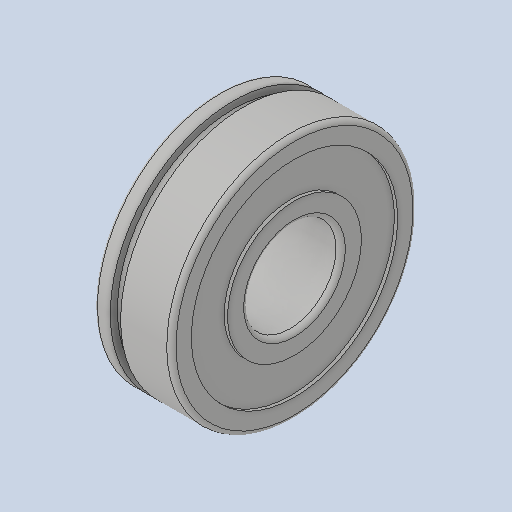
# Autodesk Inventor part: bearingB6201ZZNR
Saved by Autodesk Inventor 2025.2 (Build 292293000, 293)
## iProperties
Category: PARTsolutions
Company: MISUMI
Created: 2023-12-27
Part Number: bearingB6201ZZNR
Material: Generic
Catalog Web Link: www.cadenas.de
Description: bearing_b-Deep Groove Ball Bearings - Shield_b
Vendor: MISUMI
Document SubType Name: Modeling
Designer: psAdmin
Manufacturer: MISUMI
Mass: 6.48991 g
Surface Area: 29.9514 cm^2
Volume: 6.48991 cm^3
Density: 1 g/cm^3
Appearance: PSOLRGB-175-175-175
PSOL_IDENT_0: {$CADENAS_DATA/23d-libs/misumi/metric/12_bearing_holders/b6700zz.prj},175 {VTYP=3D},{NB=bearingB6201
PSOL_IDENT_1: ZZNR},{LINA=B6201ZZNR},{NN=bearing_b},{DATE=06.04.2023 02:22:35},{GEOMDATE=28.11.2013 13:02:00},{VER
PSOL_IDENT_2: SION=},{LINEID=100},{WBVAR=TS,TYS},{WBNUMERIC=}  {NB=bearingB6201ZZNR},{LINA=B6201ZZNR},{KT=DUMMY},{
PSOL_IDENT_3: PN=B6201ZZNR},{TS=},{TS1= '', 'Steel', 'S', 'Stainless Steel'},{TYS=NR},{TYS1=  '','w/o Retaining Ri
PSOL_IDENT_4: ng','NR','With Retaining Ring'},{MAT=52100 Bearing Steel},{BN=6201ZZ},{DD=12},{A=9.1340},{B=2.6000},
PSOL_IDENT_5: {C=2.7000},{D=32},{W=10},{RR=0.6},{CRS=6.10},{CRSS=5.78},{CORS=2.75},{CORSS=2.44},{AA=2.06},{BB=1.35
PSOL_IDENT_6: },{D1=30.15},{RR1=0.40},{RR2=0.5},{D2=36.7},{FF=1.12},{DD1=30.150},{R1=0.400},{R2=0.500},{DSMIN=16.0
PSOL_IDENT_7: },{DSMAX=17.0},{DDHH=28.0},{R=0.6},{DX=37.5},{CY=2.9},{CZ=1.2},{MASS=37},{PPATH=b6700zz_templ.prj}
NB: bearingB6201ZZNR
NN: bearing_b
NT: Deep Groove Ball Bearings - Shield_b
NBSYN: bearing$PN.
LINA: B6201ZZNR
CATALOG: Misumi
TS: Steel
TYS: With Retaining Ring
MAT: 52100 Bearing Steel
BN: 6201ZZ
DD: 12
A: 9.134
B: 2.6
C: 2.7
D: 32
W: 10
RR: 0.6
CRS: 6.10
CRSS: 5.78
CORS: 2.75
CORSS: 2.44
AA: 2.06
BB: 1.35
DD1: 30.15
R1: 0.4
R2: 0.5
DSMIN: 16
DSMAX: 17
DDHH: 28
R: 0.6
SUPPLIER: MISUMI
ARTICLENO: bearingB6201ZZNR
BOMINFO: B6201ZZNR
CREATOR: CADENAS GmbH
d2: 0.000 mm
d3: 0.000 mm
Title: B6201ZZNR
Author: Cadenas PARTsolutions
Comments: Deep Groove Ball Bearings - Shield_b
Autodesk Inventor part; units mm, degrees
sketch "Sketch_1" plane through (0, 0, 0) normal (0, 0, 1) x (1, 0, 0)
  line L0 (10, 0) -> (0, 0)
  arc A0 (0, 6.6) -> (0.6, 6) centre (0.6, 6.6) ccw
  line L1 (0.6, 6) -> (9.4, 6)
  arc A1 (9.4, 6) -> (10, 6.6) centre (9.4, 6.6) ccw
  line L2 (10, 6.6) -> (10, 8.7)
  line L3 (10, 8.7) -> (9.567, 8.7)
  line L4 (9.567, 8.7) -> (9.567, 13.4)
  line L5 (9.567, 13.4) -> (10, 13.4)
  line L6 (10, 13.4) -> (10, 15.4)
  arc A2 (10, 15.4) -> (9.4, 16) centre (9.4, 15.4) ccw
  line L7 (9.4, 16) -> (0.4, 16)
  arc A3 (0.4, 16) -> (0, 15.6) centre (0.4, 15.6) ccw
  line L8 (0, 15.6) -> (0, 13.4)
  line L9 (0, 13.4) -> (0.433, 13.4)
  line L10 (0.433, 13.4) -> (0.433, 8.7)
  line L11 (0.433, 8.7) -> (0, 8.7)
  line L12 (0, 8.7) -> (0, 6.6)
  constraints: 26 end point, 8 point on circle, 4 centre point
revolve "Revolution1" add sketch "Sketch_1" angle 360 about axis through (10, 0, 0) along (1, 0, 0)
sketch "Sketch_4" plane through (0, 0, 0) normal (0, 0, 1) x (1, 0, 0)
  line L0 (3.41, 0) -> (2.06, 0)
  line L1 (2.06, 20.075) -> (2.06, 15.075)
  line L2 (2.06, 15.075) -> (3.41, 15.075)
  line L3 (3.41, 15.075) -> (3.41, 20.075)
  line L4 (3.41, 20.075) -> (2.06, 20.075)
  constraints: 10 end point
revolve "Revolution2" cut sketch "Sketch_4" angle 360 about axis through (3.41, 0, 0) along (-1, 0, 0)
ref_plane "center_point_XY" through (5, 0, 0) normal (1, 0, 0) x (0, 0, -1)
ref_plane "center_point_YZ" through (5, 0, 0) normal (0, 0, -1) x (0, 1, 0)
ref_plane "center_point_ZX" through (5, 0, 0) normal (0, 1, 0) x (1, 0, 0)
ref_plane "to_housing_XY" through (0, 0, 0) normal (1, 0, 0) x (0, 0, -1)
ref_plane "to_housing_YZ" through (0, 0, 0) normal (0, 0, -1) x (0, 1, 0)
ref_plane "to_housing_ZX" through (0, 0, 0) normal (0, 1, 0) x (1, 0, 0)
ref_plane "to_ring_XY" through (2.06, 0, 0) normal (1, 0, 0) x (0, 0, -1)
ref_plane "to_ring_YZ" through (2.06, 0, 0) normal (0, 0, -1) x (0, 1, 0)
ref_plane "to_ring_ZX" through (2.06, 0, 0) normal (0, 1, 0) x (1, 0, 0)
body "Solid1"
